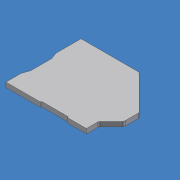
# Autodesk Inventor part: 745-500
Saved by Autodesk Inventor 2012 (Build 160160000, 160)
## iProperties
Category: PARTsolutions
Company: Team 801
Created: 2007-09-01
Part Number: 745-500
Catalog Web Link: www.team801.org
Description: 745-500 - END PLATE SNAP FIT TYPE 1.7 MM THICK
Document SubType Name: Modeling
Designer: Jeffrey M
Mass: 1.30916 g
Surface Area: 17.2897 cm^2
Volume: 1.30916 cm^3
Density: 1 g/cm^3
Material: Default
NB: 745-500
NN: 745-500
NT: END PLATE SNAP FIT TYPE 1.7 MM THICK
NBSYN: $BESTNR.
LINA: 745-500
BESTNR: 745-500
HOEHE: 27.00
BREITE: 1.70
TIEFE: 33.40
FARBE: grau
GEWICHT: 1.263
EAN: 4017332763677
RGB: 0.67,0.67,0.67,0
KT: DUMMY
PSOL_IDENT_0: {\\partserver001.servicenet\dplatte\cadenas\23d-libs\wago\pg04\serie745\0745-0500_0999-0962.prj},149
PSOL_IDENT_1: {VTYP=3D},{NB=745-500},{LINA=745-500},{NN=745-500},{DATE=24.01.2007 11:36:57},{GEOMDATE=13.06.2006}
PSOL_IDENT_2: ,{VERSION=},{LINEID=160},{LINESUBID=-1},{WBVAR=}  {NB=745-500},{LINA=745-500},{KT=DUMMY},{BESTNR=745
PSOL_IDENT_3: -500},{HOEHE=27.00},{BREITE=1.70},{TIEFE=33.40},{FARBE=grau},{GEWICHT=1.263},{EAN=4017332763677},{RG
PSOL_IDENT_4: B=0.67,0.67,0.67,0}
Title: 745-500
Author: Jeffrey M
Comments: END PLATE SNAP FIT TYPE 1.7 MM THICK
Autodesk Inventor part; units mm, degrees
ref_plane "YZ Plane" through (0, 0, 0) normal (1, 0, 0) x (0, 1, 0)
ref_plane "XZ Plane" through (0, 0, 0) normal (0, 1, 0) x (-1, 0, 0)
ref_plane "XY Plane" through (0, 0, 0) normal (0, 0, 1) x (1, 0, 0)
sketch "Skizze_1" plane through (0, 0, 0) normal (0, 0, 1) x (1, 0, 0)
  line L0 (-24.5, 0) -> (-12.2, 0)
  line L1 (-12.2, 0) -> (-12.2, 0.4)
  line L2 (-12.2, 0.4) -> (-2.6, 0.4)
  line L3 (-2.6, 0.4) -> (-2.6, 0)
  line L4 (-2.6, 0) -> (4.2, 0)
  line L5 (4.2, 0) -> (4.2, 3.9858)
  arc A0 (4.4929, 4.6929) -> (4.2, 3.9858) centre (5.2, 3.9858) ccw
  line L6 (4.4929, 4.6929) -> (8.4071, 8.6071)
  arc A1 (8.4071, 8.6071) -> (8.7, 9.3142) centre (7.7, 9.3142) ccw
  line L7 (8.7, 9.3142) -> (8.7, 13.9858)
  arc A2 (8.7, 13.9858) -> (8.4071, 14.6929) centre (7.7, 13.9858) ccw
  line L8 (8.4071, 14.6929) -> (-3.4071, 26.5071)
  arc A3 (-3.4071, 26.5071) -> (-4.1142, 26.8) centre (-4.1142, 25.8) ccw
  line L9 (-4.1142, 26.8) -> (-24.5, 26.8)
  line L10 (-24.5, 26.8) -> (-24.5, 17.8727)
  line L11 (-24.5, 17.8727) -> (-23.6, 15.4)
  line L12 (-23.6, 15.4) -> (-23.6, 7.9)
  line L13 (-23.6, 7.9) -> (-24.5, 5.4273)
  line L14 (-24.5, 5.4273) -> (-24.5, 0)
  constraints: 30 end point, 8 point on circle, 4 centre point
extrude "Extrusion1" add sketch "Skizze_1" along normal blind 1.7
body "Solid1"
